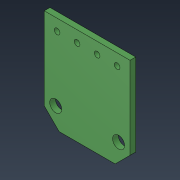
# Autodesk Inventor part: Encoderplatine
Saved by Autodesk Inventor 2022.1 (Build 261234020, 234B)
## iProperties
Part Number: Encoderplatine
Material: Phenolharz
Document SubType Name: Modeling
Designer: rYan
Density: 1.38 g/cm^3
Appearance: Glatt - waldgrün
Mass: 0.328676 g
Surface Area: 5.63057 cm^2
Volume: 0.238171 cm^3
Author: rYan
Autodesk Inventor part; units mm, degrees
ref_plane "YZ Plane" through (0, 0, 0) normal (1, 0, 0) x (0, 1, 0)
ref_plane "XZ Plane" through (0, 0, 0) normal (0, 1, 0) x (-1, 0, 0)
ref_plane "XY Plane" through (0, 0, 0) normal (0, 0, 1) x (1, 0, 0)
sketch "Skizze1" plane through (0, 0, 0) normal (0, 1, 0) x (-1, 0, 0)
  line L0 (4.9, 0) -> (-4.9, 0)
  line L1 (-4.9, 0) -> (-7.5, 2.6)
  line L2 (-7.5, 2.6) -> (-7.5, 17)
  line L3 (-7.5, 17) -> (7.5, 17)
  line L4 (7.5, 17) -> (7.5, 2.6)
  line L5 (7.5, 2.6) -> (4.9, 0)
  line L6 (0, -3.4) -> (0, 20.4) projected
  circle A0 centre (5.5, 3.6) radius 1.05
  circle A1 centre (-5.5, 3.6) radius 1.05
  point P0 (0, 0)
  dimension "d0" = 45
  dimension "d1" = 15
  dimension "d2" = 2.6
  dimension "d3" = 17
  dimension "d4" = 2.1
  dimension "d5" = 2.1
  dimension "d6" = 11
  dimension "d7" = 1
  constraints: 12 end point, 3 perpendicular, 2 centre point, 1 horizontal, 1 midpoint, 1 symmetric about line, 2 other
  measures "d0" angle of L5 L0
  measures "d1" distance of L2.end L3.end
  measures "d2" distance from line of L4.end L0
  measures "d3" distance between parallel lines of L0 L3
  measures "d4" diameter of A0
  measures "d5" diameter of A1
  measures "d6" distance of A1.centre A0.centre
  measures "d7" vertical distance of L4.end A0.centre
extrude "Extrusion1" add sketch "Skizze1" along normal blind 1
fillet "Rundung1" [suppressed]
sketch "Skizze2" plane through (0, 0, 0) normal (0, 1, 0) x (-1, 0, 0)
  line L0 (5.25, 15) -> (-5.25, 15) construction
  line L1 (0, -3) -> (0, 18) projected
  line L2 (-7.35, 0) -> (7.35, 0) projected
  point P0 (0, 0)
  point P1 (1.75, 15)
  point P2 (-1.75, 15)
  dimension "d11" = 3.5
  dimension "d12" = 3.5
  dimension "d13" = 15
  constraints: 2 coincident, 2 end point, 2 point on line, 2 symmetric about line, 1 horizontal
  measures "d11" distance of point (1.75, 15) point (5.25, 15)
  measures "d12" distance of point (-1.75, 15) point (1.75, 15)
  measures "d13" distance between parallel lines of L2 L0
hole "Bohrung1" at (1.75, 0, 15) at (-1.75, 0, 15) at (-5.25, 0, 15) at (5.25, 0, 15) direction (0, 1, 0) diameter 1 end through all
equation "\"d12\" = d11"
